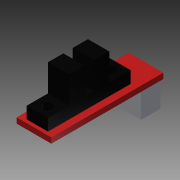
# Autodesk Inventor part: EndStopOptical
Saved by Autodesk Inventor 2016 (Build 200138000, 138)
## iProperties
Category: Electronics
Created: 2014-12-06
Part Number: EndStopOptical
Material: Generic
Document SubType Name: Modeling
Designer: Jack
Density: 1 g/cm^3
Appearance: Default
Mass: 1.88496 g
Surface Area: 16.814 cm^2
Volume: 1.88496 cm^3
Vendor: RobotDigg
Catalog Web Link: http://www.robotdigg.com/product/155/Optical-Endstop-w/-Lead-Wires-for-3D-Printers
Author: Jack
Title: End Stop Optical
Autodesk Inventor part; units mm, degrees
ref_plane "YZ Plane" through (0, 0, 0) normal (1, 0, 0) x (0, 1, 0)
ref_plane "XZ Plane" through (0, 0, 0) normal (0, 1, 0) x (-1, 0, 0)
ref_plane "XY Plane" through (0, 0, 0) normal (0, 0, 1) x (1, 0, 0)
sketch "Sketch1" plane through (0, 0, 0) normal (0, 0, 1) x (1, 0, 0)
  line L0 (0, 0) -> (10.3, 0)
  line L1 (10.3, 0) -> (10.3, 33.2)
  line L2 (10.3, 33.2) -> (0, 33.2)
  line L3 (0, 33.2) -> (0, 0)
  dimension "d0" = 10.3
  dimension "d1" = 33.2
  constraints: 8 end point, 2 parallel, 1 horizontal, 1 perpendicular
  measures "d0" distance of L2.end L1.end
  measures "d1" distance of L1.end L0.end
extrude "Extrusion1" add sketch "Sketch1" along normal blind 1.6
sketch "Sketch2" plane through (0, 0, 1.6) normal (0, 0, 1) x (1, 0, 0)
  line L0 (0, 0) -> (10.3, 0) projected
  line L1 (10.3, 0) -> (10.3, 33.2) projected
  line L2 (2, 25.5) -> (8.3, 25.5)
  line L3 (8.3, 25.5) -> (8.3, 1)
  line L4 (8.3, 1) -> (2, 1)
  line L5 (2, 1) -> (2, 25.5)
  dimension "d4" = 6.3
  dimension "d5" = 24.5
  dimension "d6" = 1
  dimension "d7" = 2
  constraints: 8 end point, 2 parallel, 1 horizontal, 1 perpendicular
  measures "d4" distance of L3.end L4.end
  measures "d5" distance of L2.end L3.end
  measures "d6" distance between parallel lines of L0 L4
  measures "d7" distance between parallel lines of L1 L3
extrude "Extrusion2" add sketch "Sketch2" along normal blind 3.5
sketch "Sketch3" plane through (0, 0, 5.1) normal (0, 0, 1) x (1, 0, 0)
  line L0 (2, 25.5) -> (2, 1) projected
  line L1 (2, 1) -> (8.3, 1) projected
  line L2 (8.3, 1) -> (8.3, 25.5) projected
  line L3 (8.3, 11.85) -> (2, 11.85)
  line L4 (2, 7.35) -> (8.3, 7.35)
  line L5 (8.3, 14.65) -> (2, 14.65)
  line L6 (2, 19.15) -> (8.3, 19.15)
  point P0 (0, 0)
  dimension "d10" = 4.5
  dimension "d11" = 4.5
  dimension "d12" = 2.8
  dimension "d13" = 10.85
  constraints: 8 end point, 8 point on line, 4 perpendicular
  measures "d10" distance between parallel lines of L5 L6
  measures "d11" distance between parallel lines of L4 L3
  measures "d12" distance between parallel lines of L3 L5
  measures "d13" distance between parallel lines of L1 L3
extrude "Extrusion3" add sketch "Sketch3" along normal blind 8 contours L6 L2 L5 L0 | L3 L2 L4 L0
sketch "Sketch4" plane through (0, 0, 0) normal (0, 0, -1) x (-1, 0, 0)
  line L0 (-10.3, 33.2) -> (0, 33.2) projected
  line L1 (-10.3, 0) -> (-10.3, 33.2) projected
  line L2 (-10.15, 32.4) -> (-0.15, 32.4)
  line L3 (-0.15, 32.4) -> (-0.15, 26.7)
  line L4 (-0.15, 26.7) -> (-10.15, 26.7)
  line L5 (-10.15, 26.7) -> (-10.15, 32.4)
  dimension "d16" = 10
  dimension "d17" = 5.7
  dimension "d18" = 0.15
  dimension "d19" = 0.8
  constraints: 8 end point, 2 parallel, 1 horizontal, 1 perpendicular
  measures "d16" distance of L3.end L4.end
  measures "d17" distance of L2.end L3.end
  measures "d18" distance between parallel lines of L1 L5
  measures "d19" distance between parallel lines of L0 L2
extrude "Extrusion4" add sketch "Sketch4" along normal blind 7.3
sketch "Sketch5" plane through (0, 0, 5.1) normal (0, 0, 1) x (1, 0, 0)
  line L0 (2, 25.5) -> (2, 19.15) projected
  line L1 (8.3, 7.35) -> (2, 7.35) projected
  line L2 (2, 7.35) -> (2, 1) projected
  line L3 (2, 1) -> (8.3, 1) projected
  line L4 (8.3, 1) -> (8.3, 7.35) projected
  circle A0 centre (5.15, 3.75) radius 1.5
  circle A1 centre (5.15, 22.75) radius 1.5
  point P0 (0, 0)
  dimension "d22" = 3
  dimension "d23" = 19
  dimension "d24" = 3.15
  dimension "d25" = 2.75
  constraints: 2 centre point, 1 equal radius, 1 vertical alignment
  measures "d22" diameter of A1
  measures "d23" distance of A1.centre A0.centre
  measures "d24" distance from line of L0 A1.centre
  measures "d25" distance from line of A0.centre L3
extrude "Extrusion5" cut sketch "Sketch5" against normal up to next contours A0 | A1
body "Solid1"
